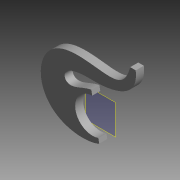
# Autodesk Inventor part: body05
Saved by Autodesk Inventor 2013 (Build 170138000, 138)
## iProperties
Created: 2013-02-19
Part Number: body05
Material: Generic
Document SubType Name: Modeling
Designer: Nano
Density: 1 g/cm^3
Author: Nano
Autodesk Inventor part; units mm, degrees
ref_plane "YZ Plane" through (0, 0, 0) normal (1, 0, 0) x (0, 1, 0)
ref_plane "XZ Plane" through (0, 0, 0) normal (0, 1, 0) x (-1, 0, 0)
ref_plane "XY Plane" through (0, 0, 0) normal (0, 0, 1) x (1, 0, 0)
ref_plane "Work Plane1" through (0, 0, -22.225) normal (0, 0, -1) x (-1, 0, 0)
sketch "Sketch1" plane through (0, 0, -22.225) normal (0, 0, -1) x (-1, 0, 0)
  arc A0 (-51.2256, -140.3966) -> (2.1978, 149.4337) centre (0, 0) ccw
  line L0 (-66.8621, -225.227) -> (19.0401, 240.8055) construction
  line L1 (-51.2256, -140.3966) -> (-58.4271, -179.4656)
  line L2 (2.1978, 149.4337) -> (9.7038, 190.1548)
  spline S0 degree 4 poles (-58.4271, -179.4656) (-17.1122, -200.4702) (128.6099, -231.8675) (412.1515, -164.2749) (492.9606, 179.0361) (260.1994, 496.1316) (-170.2187, 333.582) (-277.1446, 345.7836) (-326.0558, 527.0182) knots 0 0 0 0 0 0.207249 0.351762 0.507041 0.656346 1 1 1 1 1
  spline S1 degree 4 poles (9.7038, 190.1548) (69.4108, 178.9974) (139.3277, 136.2527) (236.7281, 109.3039) (262.2355, 236.5875) (74.6245, 280.6258) (-94.6312, 246.5021) (-374.1262, 319.7745) (-380.9677, 461.527) (-374.2103, 527.0182) knots 0 0 0 0 0 0.185379 0.30298 0.425293 0.573045 0.738735 1 1 1 1 1
  line L3 (-374.2103, 527.0182) -> (-326.0558, 527.0182)
  line L4 (-151.1409, -132.3296) -> (34.2867, -226.6016) construction
  arc A1 (-111.1953, -129.4126) -> (13.1065, -192.6081) centre (-0.5305, -65.5864) ccw construction
  line L5 (-97.3852, 210.1664) -> (116.7928, 170.1432) construction
  arc A2 (89.0312, 162.282) -> (-74.336, 192.8102) centre (-40.9173, -80.7364) ccw construction
  line L6 (-382.299, 448.6249) -> (-366.1215, 605.4116) construction
  arc A3 (-363.4012, 588.651) -> (-376.2136, 464.4769) centre (65.754, 481.6221) ccw construction
  point P0 (106.1828, -206.2675)
  point P1 (367.611, -96.7934)
  point P2 (440.7466, 164.6352)
  point P3 (288.479, 360.7138)
  point P4 (-18.3261, 379.3813)
  point P5 (226.3741, 149.4343)
  point P6 (236.7103, 200.4771)
  point P7 (130.7305, 260.0994)
  point P8 (-74.3758, 268.7935)
  point P9 (-326.0558, 360.7121)
  point P10 (164.2674, 138.3717)
  point P11 (-222.0336, 379.38)
  constraints: 14 end point, 6 midpoint, 5 point on circle, 4 centre point, 4 coincident, 4 point on line, 1 horizontal, 22 other
extrude "Extrusion1" add sketch "Sketch1" against normal blind 69.85
body "Solid1"
